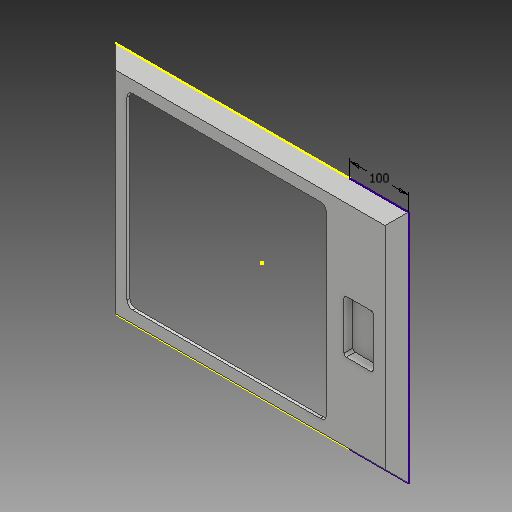
# Autodesk Inventor part: SitzFläche
Saved by Autodesk Inventor 2018 (Build 220112000, 112)
## iProperties
Created: 2019-02-06
Part Number: SitzFläche
Material: Generisch
Document SubType Name: Modeling
Designer: Lolob
Density: 1 g/cm^3
Appearance: Vorgabe
Author: Lolob
Autodesk Inventor part; units mm, degrees
ref_plane "YZ Plane" through (0, 0, 0) normal (1, 0, 0) x (0, 1, 0)
ref_plane "XZ Plane" through (0, 0, 0) normal (0, 1, 0) x (-1, 0, 0)
ref_plane "XY Plane" through (0, 0, 0) normal (0, 0, 1) x (1, 0, 0)
sketch "Skizze1" plane through (0, 0, 0) normal (0, 1, 0) x (-1, 0, 0)
  line L0 (350, 0) -> (-350, 0) projected
  line L1 (0, -280) -> (0, 280) projected
  line L2 (250, 200) -> (-250, 200)
  line L3 (-250, 200) -> (-250, -200)
  line L4 (-250, -200) -> (250, -200)
  line L5 (250, -200) -> (250, 200)
  point P0 (0, 0)
  dimension "d0" = 400
  dimension "d1" = 500
  constraints: 8 end point, 2 parallel, 1 horizontal, 1 perpendicular, 2 other
  measures "d0" distance of L2.end L3.end
  measures "d1" distance of L2.start L2.end
extrude "Extrusion1" add sketch "Skizze1" along normal blind 20
chamfer "Fase1" distance 20 angle 45 4 edges at (-250, 0, 0) (0, 0, 200) (250, 0, 0) (0, 0, -200)
sketch "Skizze2" plane through (0, 20, 0) normal (0, 1, 0) x (1, 0, 0)
  line L0 (250, -200) -> (250, 200) projected
  line L1 (250, 200) -> (-250, 200) projected
  line L2 (-250, -200) -> (250, -200) projected
  line L3 (250, 200) -> (150, 200)
  line L4 (150, 200) -> (150, -200)
  line L5 (150, -200) -> (250, -200)
  line L6 (250, -200) -> (250, 200)
  point P0 (0, 0)
  dimension "d7" = 100
  constraints: 8 end point, 2 parallel, 1 horizontal, 1 perpendicular, 1 point on line
  measures "d7" distance of L5.end L4.end
sketch "Skizze7" plane through (0, 20, 0) normal (0, 1, 0) x (1, 0, 0)
  line L0 (-250, -200) -> (250, -200) projected
  line L1 (250, -200) -> (250, 200) projected
  line L2 (250, 200) -> (-250, 200) projected
  line L3 (-250, 200) -> (-250, -200) projected
  line L4 (-350, 261.6691) -> (350, 261.6691)
  line L5 (-220, -180) -> (140, -180)
  line L6 (150, -170) -> (150, 170)
  line L7 (140, 180) -> (-220, 180)
  line L8 (-230, 170) -> (-230, -170)
  arc A0 (-230, -170) -> (-220, -180) centre (-220, -170) ccw
  arc A1 (-220, 180) -> (-230, 170) centre (-220, 170) ccw
  arc A2 (150, 170) -> (140, 180) centre (140, 170) ccw
  arc A3 (140, -180) -> (150, -170) centre (140, -170) ccw
  point P0 (0, 0)
  point P1 (458.9826, 261.6691)
  point P2 (-230, -180)
  point P3 (150, 180)
  point P4 (150, -180)
  point P5 (-230, 180)
  dimension "d35" = 380
  dimension "d37" = 20
  dimension "d38" = 20
  dimension "d41" = 10
  dimension "d53" = 20
  constraints: 10 end point, 8 point on circle, 8 point on line, 8 tangent, 4 centre point, 3 equal radius, 2 horizontal, 2 parallel, 1 perpendicular, 3 other
  measures "d35" distance of point (-230, -180) point (150, -180)
  measures "d37" distance between parallel lines of L3 L8
  measures "d38" distance between parallel lines of L0 L5
  measures "d41" radius of A0
  measures "d53" distance between parallel lines of L2 L7
extrude "Extrusion6" cut sketch "Skizze7" against normal blind 10 contours A0 L8 A1 L7 A2 L6 A3 L5
sketch "Skizze6" plane through (0, 0, 0) normal (0, -1, 0) x (1, 0, 0)
  line L0 (230, 180) -> (230, -180) projected
  line L1 (-350, 0) -> (350, 0) projected
  line L2 (160, 42.534) -> (210, 42.534)
  line L3 (210, 42.534) -> (210, -47.466)
  line L4 (210, -47.466) -> (160, -47.466)
  line L5 (160, -47.466) -> (160, 42.534)
  point P0 (0, 0)
  dimension "d23" = 50
  dimension "d24" = 90
  dimension "d25" = 20
  constraints: 8 end point, 2 parallel, 1 horizontal, 1 perpendicular
  measures "d23" distance of L2.start L2.end
  measures "d24" distance of L2.end L3.end
  measures "d25" distance between parallel lines of L0 L3
extrude "Extrusion5" cut sketch "Skizze6" against normal blind 15
fillet "Rundung1" radius 4 4 edges at (160, 7.5, 42.534) (210, 7.5, 42.534) (210, 7.5, -47.466) (160, 7.5, -47.466)
sketch "Skizze8" plane through (0, 10, 0) normal (0, 1, 0) x (1, 0, 0)
  arc A0 (140, -180) -> (150, -170) centre (140, -170) ccw projected
  line L0 (150, 170) -> (150, -170) projected
  arc A1 (150, 170) -> (140, 180) centre (140, 170) ccw projected
  arc A2 (-220, 180) -> (-230, 170) centre (-220, 170) ccw projected
  line L1 (-230, -170) -> (-230, 170) projected
  arc A3 (-230, -170) -> (-220, -180) centre (-220, -170) ccw projected
  line L2 (-220, 180) -> (140, 180) projected
  line L3 (-210, -170) -> (130, -170)
  line L4 (140, -160) -> (140, 160)
  line L5 (130, 170) -> (-210, 170)
  line L6 (-220, 160) -> (-220, -160)
  arc A4 (-220, -160) -> (-210, -170) centre (-210, -160) ccw
  arc A5 (130, -170) -> (140, -160) centre (130, -160) ccw
  arc A6 (140, 160) -> (130, 170) centre (130, 160) ccw
  arc A7 (-210, 170) -> (-220, 160) centre (-210, 160) ccw
  line L7 (140, -180) -> (-220, -180) projected
  line L8 (-220, 180) -> (140, 180) projected
  point P0 (0, 0)
  dimension "d43" = 10
  dimension "d45" = 10
  dimension "d46" = 10
  dimension "d54" = 10
  dimension "d57" = 10
  constraints: 8 end point, 8 point on circle, 8 tangent, 4 centre point, 3 equal radius, 2 parallel, 1 horizontal, 1 perpendicular
  measures "d43" distance between parallel lines of L1 L6
  measures "d45" distance between parallel lines of L0 L4
  measures "d46" radius of A4
  measures "d54" distance between parallel lines of L8 L5
  measures "d57" distance between parallel lines of L7 L3
extrude "Extrusion7" cut sketch "Skizze8" against normal blind 5 contours A4 L6 A7 L5 A6 L4 A5 L3
sketch "Skizze9" plane through (0, 5, 0) normal (0, 1, 0) x (1, 0, 0)
  line L0 (130, -170) -> (-210, -170) projected
  arc A0 (130, -170) -> (140, -160) centre (130, -160) ccw projected
  line L1 (140, 160) -> (140, -160) projected
  arc A1 (140, 160) -> (130, 170) centre (130, 160) ccw projected
  line L2 (-210, 170) -> (130, 170) projected
  arc A2 (-210, 170) -> (-220, 160) centre (-210, 160) ccw projected
  line L3 (-220, -160) -> (-220, 160) projected
  arc A3 (-220, -160) -> (-210, -170) centre (-210, -160) ccw projected
  line L4 (-200, -160) -> (120, -160)
  line L5 (130, -150) -> (130, 150)
  line L6 (120, 160) -> (-200, 160)
  line L7 (-210, 150) -> (-210, -150)
  arc A4 (-210, -150) -> (-200, -160) centre (-200, -150) ccw
  arc A5 (-200, 160) -> (-210, 150) centre (-200, 150) ccw
  arc A6 (130, 150) -> (120, 160) centre (120, 150) ccw
  arc A7 (120, -160) -> (130, -150) centre (120, -150) ccw
  point P0 (0, 0)
  dimension "d49" = 10
  constraints: 8 end point, 8 point on circle, 8 tangent, 4 centre point, 4 point on line, 3 equal radius, 2 parallel, 1 horizontal, 1 perpendicular
  measures "d49" radius of A4
extrude "Extrusion8" cut sketch "Skizze9" against normal blind 5 contours A4 L7 A5 L6 A6 L5 A7 L4
